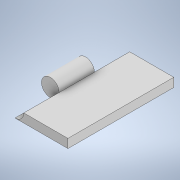
# Autodesk Inventor part: left_hinge
Saved by Autodesk Inventor 2020.3 (Build 243373000, 373)
## iProperties
Created: 2021-08-07
Part Number: left_hinge
Material: Generic
Document SubType Name: Modeling
Designer: 0x6f736f646f
Density: 1 g/cm^3
Appearance: Default
Author: 0x6f736f646f
Autodesk Inventor part; units mm, degrees
ref_plane "YZ Plane" through (0, 0, 0) normal (1, 0, 0) x (0, 1, 0)
ref_plane "XZ Plane" through (0, 0, 0) normal (0, 1, 0) x (-1, 0, 0)
sketch "Sketch1" plane through (0, 0, 0) normal (0, 0, 1) x (1, 0, 0)
  line L0 (0, 0) -> (30, 0)
  line L1 (30, 0) -> (30, 5)
  line L2 (30, 5) -> (0, 5)
  line L3 (0, 5) -> (0, 0)
  circle A0 centre (0, 5) radius 5
  point P0 (5, 5)
  dimension "d0" = 30
  dimension "d1" = 5
  dimension "d2" = 10
  dimension "d3" = 0
  constraints: 8 end point, 2 parallel, 1 centre point, 1 horizontal, 1 perpendicular, 1 tangent
  measures "d0" distance of L2.end L1.end
  measures "d1" distance of L1.end L0.end
  measures "d2" diameter of A0
  measures "d3" distance from line of A0.centre L3
extrude "Extrusion1" add sketch "Sketch1" along normal blind 60
extrude "Extrusion2" cut sketch "Sketch1" along normal blind 20 contours A0 L2 L3 | L3 L2 A0
ref_plane "Work Plane1" through (0, 0, 30) normal (0, 0, 1) x (1, 0, 0)
mirror "Mirror1" about plane through (0, 0, 30) normal (0, 0, 1) of "Extrusion2"
body "Solid1"
